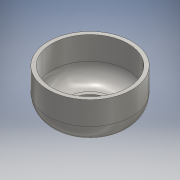
# Autodesk Inventor part: Hull
Saved by Autodesk Inventor 2016 (Build 200138000, 138)
## iProperties
Created: 2015-08-05
Part Number: Hull
Material: Generic
Document SubType Name: Modeling
Designer: 3DPrinterUser
Density: 1 g/cm^3
Appearance: Stainless - Brushed
Author: 3DPrinterUser
Autodesk Inventor part; units mm, degrees
ref_plane "YZ Plane" through (0, 0, 0) normal (1, 0, 0) x (0, 1, 0)
ref_plane "XY Plane" through (0, 0, 0) normal (0, 0, 1) x (1, 0, 0)
derived "Fixture.ipt"
sketch "Sketch1" plane through (0, 0, 0) normal (0, 1, 0) x (-1, 0, 0)
  line L0 (0, 0) -> (0, -76.5) construction
  line L1 (0, -76.5) -> (41.3, -76.5) construction
  line L2 (0, 0) -> (75.6, 0) construction
  line L3 (75.6, 0) -> (75.6, -45.99)
  line L4 (41.3, -76.5) -> (45.09, -76.5)
  arc A0 (45.09, -76.5) -> (75.6, -45.99) centre (45.09, -45.99) ccw
  line L5 (41.3, -76.5) -> (38.3, -76.5)
  line L6 (38.3, -76.5) -> (38.3, -79.5)
  line L7 (38.3, -79.5) -> (45.09, -79.5)
  arc A1 (45.09, -79.5) -> (78.6, -45.99) centre (45.09, -45.99) ccw
  line L8 (45.09, -76.5) -> (45.09, -79.5) construction
  line L9 (75.6, -45.99) -> (78.6, -45.99) construction
  line L10 (78.6, -45.99) -> (78.6, 0)
  line L11 (78.6, 0) -> (75.6, 0)
  line L12 (78.6, 0) -> (83.1, 0)
  line L13 (83.1, 0) -> (83.1, -45.99)
  arc A2 (45.09, -84) -> (83.1, -45.99) centre (45.09, -45.99) ccw
  line L14 (45.09, -84) -> (38.3, -84)
  line L15 (38.3, -84) -> (38.3, -79.5)
  dimension "d1" = 76.5
  dimension "d2" = 41.3
  dimension "d3" = 75.6
  dimension "d4" = 3
  dimension "d42" = 4.5
  constraints: 32 end point, 6 horizontal, 6 point on circle, 5 perpendicular, 5 vertical, 4 tangent, 3 centre point, 2 coincident, 1 point on line
  measures "d1" distance of L0.start L0.end
  measures "d2" distance of L0.end L1.end
  measures "d3" distance of L0.start L2.end
  measures "d4" distance of L1.end L5.end
  measures "d42" distance between parallel lines of L7 L14
revolve "Revolution1" add sketch "Sketch1" angle 360 about axis through (0, 0, 0) along (0, 0, -1)
derived "Transmission.ipt"
sketch "Sketch2" plane through (0, 0, 22.2) normal (0, 0, 1) x (1, 0, 0)
  circle A0 centre (58.4442, 0.8202) radius 25.45 construction
  circle A1 centre (0, 0) radius 75.6 construction
  circle A2 centre (58.4442, 0.8202) radius 27.45
  circle A3 centre (58.4442, 0.8202) radius 11.5 construction
  point P0 (0, 0)
  dimension "d7" = 50.9
  dimension "d11" = 2
  constraints: 2 centre point, 2 coincident
  measures "d7" diameter of A0
  measures "d11" radial gap between concentric circles of A0 A2
sketch "Sketch4" plane through (0, 0, 22.2) normal (0, 0, 1) x (1, 0, 0)
  circle A0 centre (47.4276, -34.0805) radius 1.05 construction
  circle A1 centre (53.8868, -33.3537) radius 1.05 construction
  circle A2 centre (-47.4276, 34.0805) radius 1.05 construction
  circle A3 centre (-53.8868, 33.3537) radius 1.05 construction
  arc A4 (68.319, 32.3708) -> (72.5777, 21.162) centre (70.671, 26.851) ccw construction
  arc A5 (68.319, 32.3708) -> (60.9629, 44.7089) centre (0, 0) ccw construction
  arc A6 (53.1274, 53.7851) -> (60.9629, 44.7089) centre (57.2254, 49.4026) ccw construction
  arc A7 (53.1274, 53.7851) -> (41.9951, 62.8631) centre (0, 0) ccw construction
  arc A8 (31.5279, 68.7121) -> (41.9951, 62.8631) centre (36.8776, 65.9955) ccw construction
  arc A9 (31.5279, 68.7121) -> (17.962, 73.4352) centre (0, 0) ccw construction
  arc A10 (6.1256, 75.3514) -> (17.962, 73.4352) centre (12.0818, 74.6283) ccw construction
  arc A11 (6.1256, 75.3514) -> (-8.2376, 75.1499) centre (0, 0) ccw construction
  arc A12 (-20.0156, 72.9022) -> (-8.2376, 75.1499) centre (-14.1712, 74.2599) ccw construction
  arc A13 (-20.0156, 72.9022) -> (-33.4435, 67.8004) centre (0, 0) ccw construction
  arc A14 (-43.7425, 61.66) -> (-33.4435, 67.8004) centre (-38.715, 64.9347) ccw construction
  arc A15 (-43.7425, 61.66) -> (-54.6157, 52.2731) centre (0, 0) ccw construction
  arc A16 (-62.1935, 42.9806) -> (-54.6157, 52.2731) centre (-58.5891, 47.7773) ccw construction
  arc A17 (-62.1935, 42.9806) -> (-69.2005, 30.441) centre (0, 0) ccw construction
  arc A18 (-73.143, 19.1171) -> (-69.2005, 30.441) centre (-71.3966, 24.8574) ccw construction
  arc A19 (-73.143, 19.1171) -> (-72.5777, -21.162) centre (0, 0) ccw construction
  arc A20 (-68.319, -32.3708) -> (-72.5777, -21.162) centre (-70.671, -26.851) ccw construction
  arc A21 (-68.319, -32.3708) -> (-60.9629, -44.7089) centre (0, 0) ccw construction
  arc A22 (-53.1274, -53.7851) -> (-60.9629, -44.7089) centre (-57.2254, -49.4026) ccw construction
  arc A23 (-53.1274, -53.7851) -> (-41.9951, -62.8631) centre (0, 0) ccw construction
  arc A24 (-31.5279, -68.7121) -> (-41.9951, -62.8631) centre (-36.8776, -65.9955) ccw construction
  arc A25 (-31.5279, -68.7121) -> (-17.962, -73.4352) centre (0, 0) ccw construction
  arc A26 (-6.1256, -75.3514) -> (-17.962, -73.4352) centre (-12.0818, -74.6283) ccw construction
  arc A27 (-6.1256, -75.3514) -> (8.2376, -75.1499) centre (0, 0) ccw construction
  arc A28 (20.0156, -72.9022) -> (8.2376, -75.1499) centre (14.1712, -74.2599) ccw construction
  arc A29 (20.0156, -72.9022) -> (33.4435, -67.8004) centre (0, 0) ccw construction
  arc A30 (43.7425, -61.66) -> (33.4435, -67.8004) centre (38.715, -64.9347) ccw construction
  arc A31 (43.7425, -61.66) -> (54.6157, -52.2731) centre (0, 0) ccw construction
  arc A32 (62.1935, -42.9806) -> (54.6157, -52.2731) centre (58.5891, -47.7773) ccw construction
  arc A33 (62.1935, -42.9806) -> (69.2005, -30.441) centre (0, 0) ccw construction
  arc A34 (73.143, -19.1171) -> (69.2005, -30.441) centre (71.3966, -24.8574) ccw construction
  arc A35 (73.143, -19.1171) -> (72.5777, 21.162) centre (0, 0) ccw construction
  circle A36 centre (0, 0) radius 37.3 construction
  circle A37 centre (-58.4442, -0.8201) radius 11.5 construction
  circle A38 centre (58.4442, 0.8201) radius 11.5 construction
  circle A39 centre (-70.1045, 10.5174) radius 2.7 construction
  circle A40 centre (-46.784, -12.1577) radius 2.7 construction
  circle A41 centre (69.7817, 12.4804) radius 2.7 construction
  circle A42 centre (47.1067, -10.8401) radius 2.7 construction
  circle A43 centre (70.1045, -10.5174) radius 2.7 construction
  circle A44 centre (46.784, 12.1577) radius 2.7 construction
  circle A45 centre (-47.1067, 10.8401) radius 2.7 construction
  circle A46 centre (-69.7817, -12.4804) radius 2.7 construction
  circle A47 centre (59.7811, 35.6423) radius 1.55 construction
  circle A48 centre (43.9855, 53.9392) radius 1.55 construction
  circle A49 centre (15.5523, 44.6701) radius 1.55 construction
  circle A50 centre (-0.9766, 69.5931) radius 1.55 construction
  circle A51 centre (-24.72, 65.0622) radius 1.55 construction
  circle A52 centre (-30.9093, 35.8037) radius 1.55 construction
  circle A53 centre (-60.7577, 33.9508) radius 1.55 construction
  circle A54 centre (60.7577, -33.9508) radius 1.55 construction
  circle A55 centre (45.4817, -52.6837) radius 1.55 construction
  circle A56 centre (24.72, -65.0622) radius 1.55 construction
  circle A57 centre (-40.6271, -24.2224) radius 1.55 construction
  circle A58 centre (-29.8924, -36.657) radius 1.55 construction
  circle A59 centre (-15.5523, -44.6701) radius 1.55 construction
  circle A60 centre (0.6637, -47.2953) radius 1.55 construction
  circle A61 centre (0.9766, -69.5931) radius 1.55 construction
  circle A62 centre (-22.8846, -65.7302) radius 1.55 construction
  circle A63 centre (-43.9855, -53.9392) radius 1.55 construction
  circle A64 centre (-59.7811, -35.6423) radius 1.55 construction
  circle A65 centre (16.7996, -44.2161) radius 1.55 construction
  circle A66 centre (30.9093, -35.8037) radius 1.55 construction
  circle A67 centre (41.2908, -23.0729) radius 1.55 construction
  circle A68 centre (-41.2908, 23.0729) radius 1.55 construction
  circle A69 centre (-45.4817, 52.6837) radius 1.55 construction
  circle A70 centre (-16.7996, 44.2161) radius 1.55 construction
  circle A71 centre (-0.6637, 47.2953) radius 1.55 construction
  circle A72 centre (22.8846, 65.7302) radius 1.55 construction
  circle A73 centre (29.8924, 36.657) radius 1.55 construction
  circle A74 centre (40.6271, 24.2224) radius 1.55 construction
  arc A75 (8.2376, -75.1499) -> (20.0156, -72.9022) centre (0, 0) ccw
  arc A76 (20.0156, -72.9022) -> (8.2376, -75.1499) centre (14.1712, -74.2599) ccw
  constraints: 4 point on circle, 2 centre point, 2 coincident
sketch "Sketch12" plane through (0, 83.1, -22.995) normal (0, 1, 0) x (-1, 0, 0)
  line L0 (-83.1, -22.995) -> (83.1, -22.995) projected
  line L1 (81.8521, 22.995) -> (83.1, 22.995) projected
  line L2 (0, 22.995) -> (0, -22.995) construction
  point P0 (0, 0)
  constraints: 2 end point, 2 midpoint
sketch "Sketch11" plane through (0, 0, 0) normal (1, 0, 0) x (0, 1, 0)
  line L0 (75.7, -45.99) -> (75.7, 22.2) construction
  line L1 (75.7, -32.995) -> (80.7, -32.995)
  line L2 (80.7, -32.995) -> (80.7, -12.995)
  line L3 (80.7, -12.995) -> (75.7, -12.995)
  line L4 (75.7, -12.995) -> (75.7, -32.995)
  line L5 (80.7, -22.995) -> (75.7, -22.995) construction
  line L6 (0, -59.628) -> (0, 35.838) projected
  line L7 (75.7, -23.995) -> (83.1, -23.995) construction
  line L8 (75.7, -21.995) -> (83.1, -21.995) construction
  line L9 (75.7, -21.995) -> (83.1, -21.995) projected
  line L10 (80.7, -21.995) -> (80.7, -23.995)
  line L11 (75.7, -23.995) -> (83.1, -23.995) projected
  point P0 (0, 0)
  dimension "d44" = 5
  dimension "d45" = 20
  dimension "outer_hull_radius" = 83.1
  dimension "inner_hull_diameter" = 161.4
  constraints: 12 end point, 5 point on line, 3 midpoint, 2 parallel, 1 horizontal, 1 perpendicular
sketch "Sketch8" plane through (0, 0, -84) normal (0, 0, -1) x (-1, 0, 0)
  circle A0 centre (0, 0) radius 38.4
  circle A1 centre (0, 0) radius 58.8933
  circle A2 centre (0, -48.6467) radius 4.5
  line L0 (0, -44.1467) -> (0, -38.4) construction
  circle A3 centre (0, 0) radius 38.4 construction
  line L1 (0, -53.1467) -> (0, -58.8933) construction
  circle A4 centre (0, 0) radius 58.8933 construction
  line L2 (0, -38.4) -> (0, 0) construction
  dimension "d38" = 9
  constraints: 6 end point, 4 vertical alignment, 3 vertical, 2 line through centre, 2 point on circle, 1 centre point, 1 collinear, 8 other
  measures "d38" diameter of A2
equation "\"d1\" = fixture_height + stand_height"
equation "\"d2\" = 0.5 * pvc_radius + thickness"
equation "\"d3\" = 0.5 * outer_radius"
equation "\"d4\" = thickness"
equation "\"d42\" = 1.5 * thickness"
equation "\"d7\" = transmission_diameter"
equation "\"d38\" = 3 * thickness"
equation "\"led_distance\" = 31"
equation "\"fixture_height\" = 72"
equation "\"stand_height\" = 4.5"
equation "\"pvc_radius\" = 76.6"
equation "\"thickness\" = 3"
equation "\"outer_radius\" = 151.2"
equation "\"transmission_diameter\" = 50.9"
body "Solid1"
